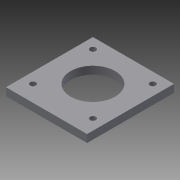
# Autodesk Inventor part: StepperHolderTop
Saved by Autodesk Inventor 2014 SP1 (Build 180222100, 222)
## iProperties
Created: 2016-11-27
Part Number: StepperHolderTop
Material: Generic
Document SubType Name: Modeling
Designer: danielsikar
Density: 1 g/cm^3
Appearance: Default
Author: danielsikar
Autodesk Inventor part; units mm, degrees
ref_plane "YZ Plane" through (0, 0, 0) normal (1, 0, 0) x (0, 1, 0)
ref_plane "XZ Plane" through (0, 0, 0) normal (0, 1, 0) x (-1, 0, 0)
ref_plane "XY Plane" through (0, 0, 0) normal (0, 0, 1) x (1, 0, 0)
sketch "Sketch1" plane through (0, 0, 0) normal (0, 0, 1) x (1, 0, 0)
  circle A0 centre (0, 0) radius 11.5
  circle A1 centre (-15.5, 15.5) radius 1.5
  circle A2 centre (-15.5, -15.5) radius 1.5
  circle A3 centre (15.5, 15.5) radius 1.5
  circle A4 centre (15.5, -15.5) radius 1.5
  line L0 (-21, -24) -> (21, -24)
  line L1 (0, 20) -> (4.5462, 20) construction
  line L2 (-21, 21) -> (-1, 21)
  line L3 (1, 21) -> (21, 21)
  line L4 (-21, 21) -> (-21, 5.9161)
  line L5 (-21, -5.9161) -> (-21, -24)
  line L6 (21, 21) -> (21, 5.9161)
  line L7 (21, -5.9161) -> (21, -24)
  line L8 (-1.865, 21) -> (1.6498, 21)
  line L9 (-21, 8.451) -> (-21, -8.8551)
  line L10 (21, 10.9387) -> (21, -8.8551)
  dimension "d0" = 23
  dimension "d1" = 3
  dimension "d2" = 3
  dimension "d3" = 24
  dimension "d4" = 8.5
  constraints: 22 end point, 6 perpendicular, 6 point on line, 5 centre point, 4 parallel, 2 horizontal, 1 coincident
  measures "d0" diameter of A0
  measures "d1" diameter of A1
  measures "d2" diameter of A2
  measures "d3" distance from line of L0 point (0, 0)
  measures "d4" distance from line of L0 A2.centre
extrude "Extrusion1" add sketch "Sketch1" along normal blind 4
body "Solid1"
